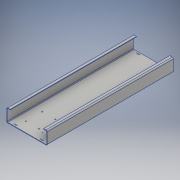
# Autodesk Inventor part: main chassis 3mm
Saved by Autodesk Inventor 2018.1 (Build 221171000, 171)
## iProperties
Created: 2018-11-28
Part Number: main chassis 3mm
Material: Aluminum 6061
Document SubType Name: Sheet Metal
Designer: RCCol
Density: 2.7 g/cm^3
Sheet Metal Rule: 3mm thick aluminum
Appearance: Aluminum - Flat
Author: RCCol
Autodesk Inventor part; units mm, degrees
ref_plane "YZ Plane" through (0, 0, 0) normal (1, 0, 0) x (0, 1, 0)
ref_plane "XZ Plane" through (0, 0, 0) normal (0, 1, 0) x (-1, 0, 0)
ref_plane "XY Plane" through (0, 0, 0) normal (0, 0, 1) x (1, 0, 0)
sketch "Sketch1" plane through (0, 0, 0) normal (0, 1, 0) x (-1, 0, 0)
  line L0 (0, 0) -> (215.9, 0)
  line L1 (215.9, 0) -> (215.9, -673.1)
  line L2 (215.9, -673.1) -> (0, -673.1)
  line L3 (0, -673.1) -> (0, 0)
  dimension "d0" = 215.9
  dimension "d1" = 673.1
  measures "d0" distance of L1.end L2.end
  measures "d1" distance of L0.end L1.end
extrude "Plate1" add sketch "Sketch1" along normal blind 3
sketch "Sketch2" plane through (-212.9, 0, 0) normal (-1, 0, 0) x (0, -1, 0)
  line L0 (0, -673.1) -> (0, 0)
  line L1 (0, 0) -> (-69.85, 0)
  line L2 (-69.85, 0) -> (-69.85, -673.1)
  line L3 (-69.85, -673.1) -> (0, -673.1)
  constraints: 6 end point, 1 horizontal, 1 perpendicular, 1 vertical
edge flange "Flange1" height 69.85 angle 90 thickness 3 bend radius 3 thickness toward (-1, 0, 0) relief straight relief width 3 relief depth 1.5 edges at (-215.9, 3, -336.55) wall of the first edge with corners at (-212.9, 0, -673.1) (-212.9, 0, 0) (-212.9, 69.85, 0) (-212.9, 69.85, -673.1)
bend "Bend1"
corner "Corner1"
sketch "Sketch3" plane through (-3, 0, -673.1) normal (1, 0, 0) x (0, 1, 0)
  line L0 (0, 673.1) -> (0, 0)
  line L1 (0, 0) -> (69.85, 0)
  line L2 (69.85, 0) -> (69.85, 673.1)
  line L3 (69.85, 673.1) -> (0, 673.1)
  constraints: 6 end point, 1 horizontal, 1 perpendicular, 1 vertical
edge flange "Flange2" height 69.85 angle 90 thickness 3 bend radius 3 thickness toward (1, 0, 0) relief straight relief width 3 relief depth 1.5 edges at (0, 3, -336.55) wall of the first edge with corners at (-3, 0, 0) (-3, 0, -673.1) (-3, 69.85, -673.1) (-3, 69.85, 0)
bend "Bend2"
corner "Corner2"
sketch "Sketch4" plane through (-215.9, 66.85, 0) normal (0, 1, 0) x (-1, 0, 0)
  line L0 (0, -673.1) -> (0, 0)
  line L1 (0, 0) -> (-19.05, 0)
  line L2 (-19.05, 0) -> (-19.05, -673.1)
  line L3 (-19.05, -673.1) -> (0, -673.1)
  constraints: 6 end point, 1 horizontal, 1 perpendicular, 1 vertical
edge flange "Flange3" height 19.05 angle 90 thickness 3 bend radius 3 thickness toward (0, 1, 0) relief straight relief width 3 relief depth 1.5 corner gap 3 corner form 0 edges at (-212.9, 69.85, -336.55) (-3, 69.85, -336.55) wall of the first edge with corners at (-215.9, 66.85, -673.1) (-215.9, 66.85, 0) (-196.85, 66.85, 0) (-196.85, 66.85, -673.1)
bend "Bend3"
corner "Corner3"
sketch "Sketch5" plane through (0, 3, 0) normal (0, 1, 0) x (1, 0, 0)
  line L0 (0, 0) -> (0, 673.3733)
  line L1 (0, 19.3233) -> (0, 654.3233)
  line L2 (-215.9, 654.3233) -> (-215.9, 19.3233)
  line L3 (-215.9, 673.3886) -> (-215.9, 0.2886)
  circle A0 centre (-41.2063, 107.0605) radius 15.1
  arc A1 (-63.0621, 108.7115) -> (-63.6574, 108.1161) centre (-63.0621, 108.1161) ccw
  arc A2 (-58.7552, 108.1161) -> (-59.3505, 108.7115) centre (-59.3505, 108.1161) ccw
  line L4 (-59.3505, 108.7115) -> (-63.0621, 108.7115)
  arc A3 (-63.6574, 106.0048) -> (-63.0621, 105.4095) centre (-63.0621, 106.0048) ccw
  line L5 (-59.3505, 105.4095) -> (-63.0621, 105.4095)
  line L6 (-63.6574, 108.1161) -> (-63.6574, 106.0048)
  line L7 (-58.7552, 108.1161) -> (-58.7552, 106.0048)
  arc A4 (-59.3505, 105.4095) -> (-58.7552, 106.0048) centre (-59.3505, 106.0048) ccw
  arc A5 (-23.0621, 108.7115) -> (-23.6574, 108.1161) centre (-23.0621, 108.1161) ccw
  arc A6 (-18.7552, 108.1161) -> (-19.3505, 108.7115) centre (-19.3505, 108.1161) ccw
  line L8 (-19.3505, 108.7115) -> (-23.0621, 108.7115)
  arc A7 (-23.6574, 106.0048) -> (-23.0621, 105.4095) centre (-23.0621, 106.0048) ccw
  line L9 (-19.3505, 105.4095) -> (-23.0621, 105.4095)
  line L10 (-23.6574, 108.1161) -> (-23.6574, 106.0048)
  line L11 (-18.7552, 108.1161) -> (-18.7552, 106.0048)
  arc A8 (-19.3505, 105.4095) -> (-18.7552, 106.0048) centre (-19.3505, 106.0048) ccw
  circle A9 centre (-68.7342, 44.746) radius 1.651
  circle A10 centre (-26.2371, 47.921) radius 1.651
  circle A11 centre (-41.2063, 171.1853) radius 15.1
  arc A12 (-63.0621, 172.8363) -> (-63.6574, 172.241) centre (-63.0621, 172.241) ccw
  arc A13 (-58.7552, 172.241) -> (-59.3505, 172.8363) centre (-59.3505, 172.241) ccw
  line L12 (-59.3505, 172.8363) -> (-63.0621, 172.8363)
  arc A14 (-63.6574, 170.1296) -> (-63.0621, 169.5343) centre (-63.0621, 170.1296) ccw
  line L13 (-59.3505, 169.5343) -> (-63.0621, 169.5343)
  line L14 (-63.6574, 172.241) -> (-63.6574, 170.1296)
  line L15 (-58.7552, 172.241) -> (-58.7552, 170.1296)
  arc A15 (-59.3505, 169.5343) -> (-58.7552, 170.1296) centre (-59.3505, 170.1296) ccw
  arc A16 (-23.0621, 172.8363) -> (-23.6574, 172.241) centre (-23.0621, 172.241) ccw
  arc A17 (-18.7552, 172.241) -> (-19.3505, 172.8363) centre (-19.3505, 172.241) ccw
  line L16 (-19.3505, 172.8363) -> (-23.0621, 172.8363)
  arc A18 (-23.6574, 170.1296) -> (-23.0621, 169.5343) centre (-23.0621, 170.1296) ccw
  line L17 (-19.3505, 169.5343) -> (-23.0621, 169.5343)
  line L18 (-23.6574, 172.241) -> (-23.6574, 170.1296)
  line L19 (-18.7552, 172.241) -> (-18.7552, 170.1296)
  arc A19 (-19.3505, 169.5343) -> (-18.7552, 170.1296) centre (-19.3505, 170.1296) ccw
  circle A20 centre (-26.2371, 139.3355) radius 1.651
  circle A21 centre (-41.2063, 230.3076) radius 9.525
  circle A22 centre (-25.3313, 230.3076) radius 1.651
  circle A23 centre (-57.0813, 230.3076) radius 1.651
  circle A24 centre (-41.2063, 268.4076) radius 9.525
  circle A25 centre (-25.3313, 268.4076) radius 1.651
  circle A26 centre (-57.0813, 268.4076) radius 1.651
  circle A27 centre (-41.2063, 306.5076) radius 9.525
  circle A28 centre (-25.3313, 306.5076) radius 1.651
  circle A29 centre (-57.0813, 306.5076) radius 1.651
  circle A30 centre (-41.2063, 354.1326) radius 15
  circle A31 centre (-41.2063, 401.7576) radius 9.525
  circle A32 centre (-25.3313, 401.7576) radius 1.651
  circle A33 centre (-57.0813, 401.7576) radius 1.651
  circle A34 centre (-41.2063, 562.0329) radius 9.525
  circle A35 centre (-25.3313, 562.0329) radius 1.651
  circle A36 centre (-57.0813, 562.0329) radius 1.651
  circle A37 centre (-41.2063, 606.4829) radius 9.525
  circle A38 centre (-25.3313, 606.4829) radius 1.651
  circle A39 centre (-57.0813, 606.4829) radius 1.651
  line L20 (-215.9, 0.2886) -> (0, 0)
  line L21 (-215.9, 673.3886) -> (0, 673.3733)
  line L22 (-162.9682, 65.2973) -> (-162.9682, 129.0513)
  arc A40 (-155.0942, 136.9253) -> (-162.9682, 129.0513) centre (-155.0942, 129.0513) ccw
  line L23 (-155.0942, 136.9253) -> (-108.3582, 136.9253)
  arc A41 (-100.4842, 129.0513) -> (-108.3582, 136.9253) centre (-108.3582, 129.0513) ccw
  line L24 (-100.4842, 129.0513) -> (-100.4842, 65.2973)
  arc A42 (-108.3582, 57.4233) -> (-100.4842, 65.2973) centre (-108.3582, 65.2973) ccw
  line L25 (-108.3582, 57.4233) -> (-155.0942, 57.4233)
  arc A43 (-162.9682, 65.2973) -> (-155.0942, 57.4233) centre (-155.0942, 65.2973) ccw
  circle A44 centre (-96.8012, 53.4863) radius 2.7813
  circle A45 centre (-96.8012, 140.8623) radius 2.7813
  circle A46 centre (-166.6512, 53.4863) radius 2.7813
  circle A47 centre (-166.6512, 140.8623) radius 2.7813
  circle A48 centre (-41.2063, 498.5329) radius 15.1
  arc A49 (-63.0621, 500.1839) -> (-63.6574, 499.5886) centre (-63.0621, 499.5886) ccw
  arc A50 (-58.7552, 499.5886) -> (-59.3505, 500.1839) centre (-59.3505, 499.5886) ccw
  line L26 (-59.3505, 500.1839) -> (-63.0621, 500.1839)
  arc A51 (-63.6574, 497.4772) -> (-63.0621, 496.8819) centre (-63.0621, 497.4772) ccw
  line L27 (-59.3505, 496.8819) -> (-63.0621, 496.8819)
  line L28 (-63.6574, 499.5886) -> (-63.6574, 497.4772)
  line L29 (-58.7552, 499.5886) -> (-58.7552, 497.4772)
  arc A52 (-59.3505, 496.8819) -> (-58.7552, 497.4772) centre (-59.3505, 497.4772) ccw
  arc A53 (-23.0621, 500.1839) -> (-23.6574, 499.5886) centre (-23.0621, 499.5886) ccw
  arc A54 (-18.7552, 499.5886) -> (-19.3505, 500.1839) centre (-19.3505, 499.5886) ccw
  line L30 (-19.3505, 500.1839) -> (-23.0621, 500.1839)
  arc A55 (-23.6574, 497.4772) -> (-23.0621, 496.8819) centre (-23.0621, 497.4772) ccw
  line L31 (-19.3505, 496.8819) -> (-23.0621, 496.8819)
  line L32 (-23.6574, 499.5886) -> (-23.6574, 497.4772)
  line L33 (-18.7552, 499.5886) -> (-18.7552, 497.4772)
  arc A56 (-19.3505, 496.8819) -> (-18.7552, 497.4772) centre (-19.3505, 497.4772) ccw
  circle A57 centre (-30.7594, 663.8483) radius 1.5875
  circle A58 centre (-185.1406, 663.8483) radius 1.5875
  circle A59 centre (-177.8, 663.8483) radius 2.667
  circle A60 centre (-170.4594, 663.8483) radius 1.5875
  circle A61 centre (-45.4406, 663.8483) radius 1.5875
  circle A62 centre (-38.1, 663.8483) radius 2.667
  circle A63 centre (-185.1406, 9.6617) radius 1.5875
  circle A64 centre (-177.8, 9.6617) radius 2.667
  circle A65 centre (-170.4594, 9.6617) radius 1.5875
  circle A66 centre (-45.4406, 9.6617) radius 1.5875
  circle A67 centre (-38.1, 9.6617) radius 2.667
  circle A68 centre (-30.7594, 9.6617) radius 1.5875
  constraints: 69 centre point, 68 end point, 56 point on circle
extrude "Cut1" cut sketch "Sketch5" against normal blind 3 contours A0 | A9 | A10 | A11 | A20 | A21 | A22 | A23 | A24 | A25 | A26 | A27 | A28 | A29 | A30 | A31 | A32 | A33 | A34 | A35 | A36 | A37 | A38 | A39 | A44 | A45 | A46 | A47 | A48 | A57 | A58 | A59 | A60 | A61 | A62 | A63 | A64 | A65 | A66 | A67 | A68
equation "\"d33\" = Thickness"
equation "\"d2\" = Thickness"
equation "\"d3\" = BendReliefWidth"
equation "\"d4\" = BendReliefDepth"
equation "\"d5\" = MinimumRemnant"
equation "\"d6\" = TransitionRadius"
equation "\"d9\" = BendRadius"
equation "\"d10\" = CornerReliefSize"
equation "\"d11\" = GapSize"
equation "\"d12\" = JacobiRadiusSize"
equation "\"d13\" = BendReliefWidth"
equation "\"d14\" = BendReliefDepth"
equation "\"d15\" = MinimumRemnant"
equation "\"d16\" = TransitionRadius"
equation "\"d19\" = BendRadius"
equation "\"d20\" = CornerReliefSize"
equation "\"d21\" = GapSize"
equation "\"d22\" = JacobiRadiusSize"
equation "\"d23\" = BendReliefWidth"
equation "\"d24\" = BendReliefDepth"
equation "\"d25\" = MinimumRemnant"
equation "\"d26\" = TransitionRadius"
equation "\"d29\" = BendRadius"
equation "\"d30\" = CornerReliefSize"
equation "\"d31\" = GapSize"
equation "\"d32\" = JacobiRadiusSize"
equation "\"BendRadius\" = Thickness"
equation "\"BendReliefWidth\" = Thickness"
equation "\"BendReliefDepth\" = 0.5 * Thickness"
equation "\"CornerReliefSize\" = 4 * Thickness"
equation "\"MinimumRemnant\" = 2 * Thickness"
equation "\"TransitionRadius\" = BendRadius"
equation "\"JacobiRadiusSize\" = BendRadius"
equation "\"GapSize\" = Thickness"
equation "\"Thickness\" = 3"
body "Solid1"
